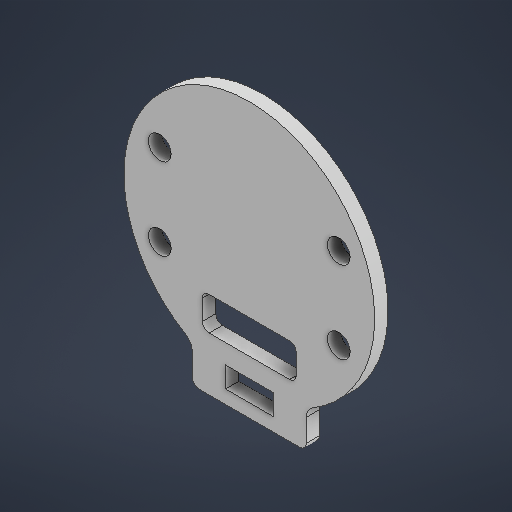
# Autodesk Inventor part: Držák-Disp
Saved by Autodesk Inventor 2026 (Build 300175000, 175)
## iProperties
Created: 2025-06-20
Part Number: Držák-Disp
Material: Všeobecné
Document SubType Name: Modeling
Designer: vadim
Density: 1 g/cm^3
Appearance: Výchozí
Author: vadim
Autodesk Inventor part; units mm, degrees
ref_plane "YZ Plane" through (0, 0, 0) normal (1, 0, 0) x (0, 1, 0)
ref_plane "XZ Plane" through (0, 0, 0) normal (0, 1, 0) x (-1, 0, 0)
ref_plane "XY Plane" through (0, 0, 0) normal (0, 0, 1) x (1, 0, 0)
sketch "Náčrt1" plane through (0, 0, 0) normal (0, 0, 1) x (1, 0, 0)
  arc A0 (8.5, -16.6565) -> (-8.5, -16.6565) centre (0, 0) ccw
  line L0 (8.5, -16.6565) -> (8.5, -22.2)
  line L1 (8.5, -22.2) -> (-8.5, -22.2)
  line L2 (-8.5, -22.2) -> (-8.5, -16.6565)
  line L3 (0, -18.7455) -> (8.5, -22.2) construction
  line L4 (0, -18.7455) -> (-8.5, -22.2) construction
  line L5 (0, 18.7) -> (0, -18.7455)
  line L6 (-13.35, 6.1) -> (13.35, 6.1)
  line L7 (13.35, 6.1) -> (13.35, -6.1)
  line L8 (13.35, -6.1) -> (-13.35, -6.1)
  line L9 (-13.35, -6.1) -> (-13.35, 6.1)
  line L10 (-13.35, 6.1) -> (13.35, -6.1) construction
  line L11 (13.35, 6.1) -> (-13.35, -6.1) construction
  circle A1 centre (-13.35, 6.1) radius 2.75
  circle A2 centre (-13.35, 6.1) radius 1.7
  circle A3 centre (-13.35, -6.1) radius 2.75
  circle A4 centre (-13.35, -6.1) radius 1.7
  circle A5 centre (13.35, -6.1) radius 2.75
  circle A6 centre (13.35, -6.1) radius 1.7
  circle A7 centre (13.35, 6.1) radius 2.75
  circle A8 centre (13.35, 6.1) radius 1.7
  line L12 (-7, -9.2) -> (7, -9.2)
  line L13 (7, -9.2) -> (7, -14.2)
  line L14 (7, -14.2) -> (-7, -14.2)
  line L15 (-7, -14.2) -> (-7, -9.2)
  line L16 (-7, -9.2) -> (7, -14.2) construction
  line L17 (7, -9.2) -> (-7, -14.2) construction
  line L18 (-3.55, -20.2) -> (3.55, -20.2)
  line L19 (3.55, -20.2) -> (3.55, -17.1)
  line L20 (3.55, -17.1) -> (-3.55, -17.1)
  line L21 (-3.55, -17.1) -> (-3.55, -20.2)
  line L22 (-3.55, -20.2) -> (3.55, -17.1) construction
  line L23 (3.55, -20.2) -> (-3.55, -17.1) construction
  point P0 (0, -11.7)
  point P1 (0, -18.65)
  point P2 (7, -6.1)
  point P3 (-7, -6.1)
  dimension "d0" = 37.4
  dimension "d1" = 17
  dimension "d2" = 22.2
  dimension "d3" = 26.7
  dimension "d4" = 12.2
  dimension "d5" = 5.5
  dimension "d6" = 3.4
  dimension "d7" = 5.5
  dimension "d8" = 3.4
  dimension "d9" = 5.5
  dimension "d10" = 3.4
  dimension "d11" = 5.5
  dimension "d12" = 3.4
  dimension "d15" = 14
  dimension "d16" = 5
  dimension "d21" = 7.1
  dimension "d22" = 3.1
  dimension "d23" = 2
  dimension "d24" = 8
  constraints: 48 end point, 9 centre point, 9 coincident, 8 parallel, 6 midpoint, 4 perpendicular, 3 horizontal, 3 point on circle, 2 point on line, 1 vertical, 2 other
  measures "d0" diameter of A0
  measures "d1" distance of L0.end L1.end
  measures "d2" distance from line of L1 A0.centre
  measures "d3" distance of L7.end L8.end
  measures "d4" distance of L6.end L7.end
  measures "d5" diameter of A1
  measures "d6" diameter of A2
  measures "d7" diameter of A3
  measures "d8" diameter of A4
  measures "d9" diameter of A5
  measures "d10" diameter of A6
  measures "d11" diameter of A7
  measures "d12" diameter of A8
  measures "d15" distance of L13.end L14.end
  measures "d16" distance of L12.end L13.end
  measures "d21" distance of L20.end L19.end
  measures "d22" distance of L19.end L18.end
  measures "d23" distance between parallel lines of L1 L18
  measures "d24" distance between parallel lines of L1 L14
extrude "Vysunutí1" add sketch "Náčrt1" along normal blind 2 contours L6 A7 L7 A5 L8 L5 | L5 L8 A3 L9 A1 L6 | L0 L1 L2 A0 | A1 L9 A2 L6 | L6 A2 L9 A1 | A7 L7 A8 L6 | L6 A8 L7 A7 | A5 L7 A6 L8 | L8 A6 L7 A5 | A3 L9 A4 L8 | L8 A4 L9 A3
fillet "Zaoblení1" radius 2 2 edges at (-8.5, -16.6565, 1) (8.5, -16.6565, 1)
fillet "Zaoblení2" radius 1 2 edges at (8.5, -22.2, 1) (-8.5, -22.2, 1)
fillet "Zaoblení3" radius 1 4 edges at (-7, -9.2, 1) (7, -9.2, 1) (-7, -14.2, 1) (7, -14.2, 1)
